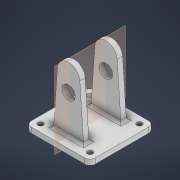
# Autodesk Inventor part: SUSPENSION_MOUNTING_BRACKET(INCOMPLETE)
Saved by Autodesk Inventor 2022 (Build 260153000, 153)
## iProperties
Created: 2024-03-05
Part Number: SUSPENSION_MOUNTING_BRACKET(INCOMPLETE)
Material: Generic
Document SubType Name: Modeling
Designer: Todd McKenzie
Density: 1 g/cm^3
Appearance: Default
Author: Todd McKenzie
Autodesk Inventor part; units mm, degrees
ref_plane "YZ Plane" through (0, 0, 0) normal (1, 0, 0) x (0, 1, 0)
ref_plane "XZ Plane" through (0, 0, 0) normal (0, 1, 0) x (-1, 0, 0)
ref_plane "XY Plane" through (0, 0, 0) normal (0, 0, 1) x (1, 0, 0)
sketch "Sketch1" plane through (0, 0, 0) normal (0, 1, 0) x (-1, 0, 0)
  line L0 (38.1, -38.1) -> (-38.1, -38.1)
  line L1 (-38.1, -38.1) -> (-38.1, 38.1)
  line L2 (-38.1, 38.1) -> (38.1, 38.1)
  line L3 (38.1, 38.1) -> (38.1, -38.1)
  line L4 (0, 0) -> (52.4018, 0)
  dimension "d0" = 76.2
  dimension "d1" = 76.2
  dimension "d2" = 38.1
  dimension "d4" = 38.1
  constraints: 10 end point, 2 horizontal, 2 parallel, 1 perpendicular
  measures "d0" distance of L2.end L0.start
  measures "d1" distance of L0.start L0.end
  measures "d2" distance from line of L3 L4.start
  measures "d4" distance between parallel lines of L2 L4
extrude "Extrusion1" add sketch "Sketch1" along normal blind 6.35
fillet "Fillet1" radius 6.35 4 edges at (38.1, 3.175, 38.1) (38.1, 3.175, -38.1) (-38.1, 3.175, 38.1) (-38.1, 3.175, -38.1)
sketch "Sketch2" plane through (0, 6.35, 0) normal (0, 1, 0) x (1, 0, 0)
  line L0 (-38.1, 31.75) -> (-38.1, -31.75) projected
  line L1 (-31.75, -38.1) -> (31.75, -38.1) projected
  point P0 (0, 0)
  point P1 (-29.3624, -29.3624)
  dimension "d15" = 8.7376
  dimension "d16" = 8.7376
  measures "d15" distance from line of L0 point (-29.362, -29.362)
  measures "d16" distance from line of L1 point (-29.362, -29.362)
hole "Hole1" at (-29.3624, 6.35, 29.3624) direction (0, -1, 0) diameter 6.35 end through all
pattern_linear "Rectangular Pattern1" count 2 spacing 58.7248 along (1, 0, 0) count 2 spacing 58.7248 along (0, 0, -1) of "Hole1"
sketch "Sketch3" plane through (0, 6.35, 0) normal (0, 1, 0) x (1, 0, 0)
  line L0 (0, 25.4) -> (-17.78, 25.4)
  line L1 (-17.78, 25.4) -> (-17.78, 0)
  line L2 (-17.78, 0) -> (-17.78, -25.4)
  line L3 (-17.78, -25.4) -> (0, -25.4)
  line L4 (0, -25.4) -> (17.78, -25.4)
  line L5 (17.78, -25.4) -> (17.78, 0)
  line L6 (17.78, 0) -> (17.78, 25.4)
  line L7 (0, 25.4) -> (17.78, 25.4)
  line L8 (0, 20.6698) -> (0, -20.9969)
  line L9 (7.902, 0) -> (-15.4374, 0)
  line L10 (7.902, 0) -> (18.1893, 0)
  line L11 (31.75, 38.1) -> (-31.75, 38.1) projected
  line L12 (-31.75, -38.1) -> (31.75, -38.1) projected
  line L13 (38.1, -31.75) -> (38.1, 31.75) projected
  line L14 (-38.1, 31.75) -> (-38.1, -31.75) projected
  point P0 (0, 0)
  dimension "d26" = 12.7
  dimension "d28" = 12.7
  dimension "d29" = 20.32
  dimension "d30" = 20.32
  constraints: 22 end point, 4 perpendicular, 4 point on line, 3 horizontal, 1 vertical
  measures "d26" distance between parallel lines of L11 L0
  measures "d28" distance between parallel lines of L3 L12
  measures "d29" distance between parallel lines of L13 L6
  measures "d30" distance between parallel lines of L14 L1
extrude "Extrusion2" add sketch "Sketch3" along normal blind 76.2
sketch "Sketch4" plane through (-17.78, 6.35, 25.4) normal (0, 0, 1) x (1, 0, 0)
  line L0 (0, 0) -> (31.3329, 0)
  line L1 (49.53, 0) -> (-13.97, 0) projected
  line L2 (0, 76.2) -> (35.56, 76.2) projected
  arc A0 (21.8819, 71.0504) -> (9.3513, 70.6828) centre (15.6464, 69.85) ccw
  line L3 (0, 0) -> (0, 76.2) projected
  line L4 (35.56, 0) -> (35.56, 76.2) projected
  line L5 (9.3513, 70.6828) -> (0, 0)
  line L6 (21.8819, 71.0504) -> (35.56, 0)
  line L7 (0, 0) -> (0, 76.2)
  line L8 (0, 76.2) -> (35.56, 76.2)
  line L9 (35.56, 76.2) -> (35.56, 0)
  point P0 (17.78, -6.35)
  point P1 (15.6464, 76.2)
  dimension "d41" = 6.35
  dimension "d47" = 15.6464
  dimension "d48" = 19.9136
  constraints: 12 end point, 2 point on circle, 2 point on line, 2 tangent, 1 centre point, 1 collinear, 1 perpendicular
  measures "d41" radius of A0
  measures "d47" distance from line of A0.centre L3
  measures "d48" distance from line of A0.centre L4
extrude "Extrusion3" [suppressed]
ref_plane "Work Plane2" through (0, 0, 31.75) normal (1, 0, 0) x (0, 0, -1)
sketch "Sketch8" plane through (0, 0, 31.75) normal (1, 0, 0) x (0, 0, -1)
  line L0 (47.9295, 82.55) -> (15.5705, 82.55) projected
  line L1 (22.7623, 82.55) -> (40.8618, 82.55)
  line L2 (15.5705, 6.35) -> (47.9295, 6.35) projected
  line L3 (40.8618, 6.35) -> (40.8618, 82.55)
  line L4 (22.7623, 82.55) -> (22.7623, 6.35)
  line L5 (22.7623, 6.35) -> (40.8618, 6.35)
  point P0 (31.75, 0)
  point P1 (22.7623, 6.35)
  constraints: 8 end point, 3 point on line, 2 perpendicular, 1 vertical
extrude "Extrusion4" [suppressed]
sketch "Sketch9" plane through (17.78, 6.35, -25.4) normal (0, 0, -1) x (-1, 0, 0)
  line L0 (17.78, -6.35) -> (17.78, 45.0353)
  circle A0 centre (17.78, 45.0353) radius 7.9375
  dimension "d59" = 51.3853
  dimension "d60" = 15.875
  constraints: 2 end point, 1 centre point, 1 coincident, 1 vertical
  measures "d59" distance of L0.start L0.end
  measures "d60" diameter of A0
sketch "Sketch10" plane through (17.78, 6.35, -25.4) normal (0, 0, -1) x (-1, 0, 0)
  point P0 (17.78, -6.35)
sketch "Sketch11" plane through (17.78, 6.35, -25.4) normal (0, 0, -1) x (-1, 0, 0)
  line L0 (0, 0) -> (0, 76.2) projected
  line L1 (0, 0) -> (4.4777, 63.7986)
  line L2 (0, 0) -> (35.56, 0) projected
  line L3 (35.56, 0) -> (31.0823, 63.7986)
  arc A0 (31.0823, 63.7986) -> (4.4777, 63.7986) centre (17.78, 62.865) ccw
  line L4 (0, 76.2) -> (35.56, 76.2) projected
  line L5 (35.56, 0) -> (35.56, 76.2) projected
  line L6 (0, 0) -> (35.56, 0)
  point P0 (17.78, -6.35)
  point P1 (17.78, 76.2)
  dimension "d61" = 13.335
  constraints: 6 end point, 3 tangent, 2 point on circle, 1 centre point, 1 equal length, 1 perpendicular
  measures "d61" radius of A0
extrude "Extrusion5" cut sketch "Sketch11" against normal blind 50.8 contours L0 L4 A0 L1 | L3 A0 L4 L5
extrude "Extrusion6" cut sketch "Sketch9" against normal blind 50.8
fillet "Fillet3" radius 3.175 4 edges at (17.78, 6.35, 0) (0, 6.35, -25.4) (-17.78, 6.35, 0) (0, 6.35, 25.4)
sketch "Sketch15" plane through (0, 0, 31.75) normal (1, 0, 0) x (0, 0, -1)
  line L0 (6.35, 82.55) -> (57.15, 82.55) projected
  line L1 (12.7, 82.55) -> (12.7, 6.35)
  line L2 (0, 6.35) -> (63.5, 6.35) projected
  line L3 (12.7, 82.55) -> (50.8, 82.55)
  line L4 (50.8, 82.55) -> (50.8, 6.35)
  line L5 (50.8, 6.35) -> (12.7, 6.35)
  line L6 (6.35, 82.55) -> (6.35, 70.1486) projected
  line L7 (57.15, 70.1486) -> (57.15, 82.55) projected
  point P0 (31.75, 0)
  point P1 (50.8, 6.35)
  dimension "d71" = 38.1
  dimension "d72" = 6.35
  dimension "d73" = 6.35
  constraints: 8 end point, 2 perpendicular, 2 point on line, 1 horizontal, 1 vertical
  measures "d71" distance between parallel lines of L4 L1
  measures "d72" distance between parallel lines of L1 L6
  measures "d73" distance between parallel lines of L7 L4
extrude "Extrusion7" cut sketch "Sketch15" along normal mid plane 50.8
fillet "Fillet4" radius 3.175 2 edges at (0, 6.35, 19.05) (0, 6.35, -19.05)
equation "\"d28\" = d26"
equation "\"d30\" = d29"
body "Solid1"
